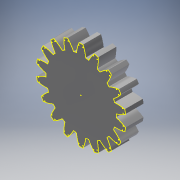
# Autodesk Inventor part: Цилиндрическое зубчатое зацепление1
Saved by Autodesk Inventor 2019 (Build 230136000, 136)
## iProperties
Created: 2020-02-27
Part Number: Цилиндрическое зубчатое зацепление1
Material: Steel
Document SubType Name: Modeling
Designer: Петров Иван
Categories: <?xml version="1.0" encoding="UTF-16"?> <MemberInstance><Categories><FamilyTemplate><FamilyTemplateParameter ValueType="xs:double" Id="1" ObjectReferenceKey="da_z" ObjectType="kUserParameterObject"/><FamilyTemplateParameter ValueType="xs:double" Id="2" ObjectReferenceKey="da_b" ObjectType="kUserParameterObject"/><FamilyTemplateParameter ValueType="xs:double" Id="3" ObjectReferenceKey="da_beta" ObjectType="kUserParameterObject"/><FamilyTemplateParameter ValueType="xs:double" Id="4" ObjectReferenceKey="da_da" ObjectType="kUserParameterObject"/><FamilyTemplateParameter ValueType="xs:double" Id="5" ObjectReferenceKey="da_aw" ObjectType="kUserParameterObject"/><FamilyTemplateParameter ValueType="xs:string" Id="6" ObjectReferenceKey="EAIAABAAAACIAQAAAAAAAIAAAAAAAAAA" ObjectType="83910656" SubObjectId="SurfaceGeometry"/></FamilyTemplate><ParamToTemplateMap><ParamToTemplate CategoryParameter="//CategoryParameter[@InternalName='046C89C9-8512-4d59-83FE-43B91F4F132A']" TemplateParameter="1"/><ParamToTemplate CategoryParameter="//CategoryParameter[@InternalName='2552DF32-E462-4b46-AEBF-C6C7768E72AC']" TemplateParameter="2"/><ParamToTemplate CategoryParameter="//CategoryParameter[@InternalName='C9EE641D-15FC-4fae-A226-E94C4372FDD7']" TemplateParameter="3"/><ParamToTemplate><ParamToTemplate CategoryParameter="//CategoryParameter[@InternalName='00B6519A-459B-49c7-AD84-2E56D39A5744']" ConstantValue="0.000000"/></ParamToTemplate><ParamToTemplate><ParamToTemplate CategoryParameter="//CategoryParameter[@InternalName='04B31F0E-C7A6-4894-AA32-9629BEFACF47']" ConstantValue="1.000000"/></ParamToTemplate><ParamToTemplate><ParamToTemplate CategoryParameter="//CategoryParameter[@InternalName='43CBEC2E-7847-49e7-A936-2F7889FCB2D9']" ConstantValue="0.250000"/></ParamToTemplate><ParamToTemplate><ParamToTemplate CategoryParameter="//CategoryParameter[@InternalName='B1EFC894-105D-4ebd-86BF-FA20ED196853']" ConstantValue="0.350000"/></ParamToTemplate><ParamToTemplate><ParamToTemplate CategoryParameter="//CategoryParameter[@InternalName='51175063-3D10-4879-93E8-6246FE8B403D']" ConstantValue="2060000000.000000"/></ParamToTemplate><ParamToTemplate><ParamToTemplate CategoryParameter="//CategoryParameter[@InternalName='A3A52E27-4454-46a9-B0BD-C932399B70AF']" ConstantValue="0.300000"/></ParamToTemplate><ParamToTemplate><ParamToTemplate CategoryParameter="//CategoryParameter[@InternalName='91B76062-C214-41d9-B1B9-14D2AB99603D']" ConstantValue="0.175000"/></ParamToTemplate><ParamToTemplate><ParamToTemplate CategoryParameter="//CategoryParameter[@InternalName='374E806E-8B8A-4dda-A9AA-1039D6500AD2']" ConstantValue="5.714286"/></ParamToTemplate><ParamToTemplate><ParamToTemplate CategoryParameter="//CategoryParameter[@InternalName='2D373A89-B862-43d6-8D0B-0CBF12AB9F6C']" ConstantValue="0.523599"/></ParamToTemplate><ParamToTemplate CategoryParameter="//CategoryParameter[@InternalName='37777632-D6A2-4fac-9D53-DB8ACD95C989']" TemplateParameter="4"/><ParamToTemplate CategoryParameter="//CategoryParameter[@InternalName='FD1017F1-B727-4f7e-9707-0F86F1FF9423']" TemplateParameter="5"/><ParamToTemplate><ParamToTemplate CategoryParameter="//CategoryParameter[@InternalName='9E1B4470-B2D3-4ff1-B813-535BB4CDF51A']" ConstantValue="3520000.000000"/></ParamToTemplate><ParamToTemplate><ParamToTemplate CategoryParameter="//CategoryParameter[@InternalName='F8452263-BFF6-458c-9FB1-07C4B99E95CD']" ConstantValue="11400000.000000"/></ParamToTemplate><ParamToTemplate><ParamToTemplate CategoryParameter="//CategoryParameter[@InternalName='3E3BB259-FD49-497f-8171-6EBC954A3479']" ConstantValue="2.000000"/></ParamToTemplate><ParamToTemplate CategoryParameter="//CategoryParameter[@InternalName='27C3BAF2-7550-4e4b-AE2C-0DB134B7D9B7']" TemplateParameter="6"/></ParamToTemplateMap><Category DisplayName="Gear" InternalName="DC85795E-93AB-48d5-8EEE-5A27447B64BD" Mnemonic="Gear"><CategoryParameter DisplayName="z" InternalName="046C89C9-8512-4d59-83FE-43B91F4F132A" Mnemonic="z"/><CategoryParameter DisplayName="b" InternalName="2552DF32-E462-4b46-AEBF-C6C7768E72AC" Mnemonic="b"/><CategoryParameter DisplayName="||b|" InternalName="C9EE641D-15FC-4fae-A226-E94C4372FDD7" Mnemonic="beta"/><CategoryParameter DisplayName="x" InternalName="00B6519A-459B-49c7-AD84-2E56D39A5744" Mnemonic="x"/><CategoryParameter DisplayName="a*" InternalName="04B31F0E-C7A6-4894-AA32-9629BEFACF47" Mnemonic="a"/><CategoryParameter DisplayName="c*" InternalName="43CBEC2E-7847-49e7-A936-2F7889FCB2D9" Mnemonic="c"/><CategoryParameter DisplayName="r|.f|*" InternalName="B1EFC894-105D-4ebd-86BF-FA20ED196853" Mnemonic="rf"/><CategoryParameter DisplayName="E" InternalName="51175063-3D10-4879-93E8-6246FE8B403D" Mnemonic="E"/><CategoryParameter DisplayName="||m|" InternalName="A3A52E27-4454-46a9-B0BD-C932399B70AF" Mnemonic="mi"/><Category DisplayName="SpurGear" InternalName="26C5A22E-A91E-4dfd-A3B3-23CCAFAE1764" Mnemonic="SpurGear"><CategoryParameter DisplayName="m" InternalName="91B76062-C214-41d9-B1B9-14D2AB99603D" Mnemonic="m"/><CategoryParameter DisplayName="P" InternalName="374E806E-8B8A-4dda-A9AA-1039D6500AD2" Mnemonic="PP"/><CategoryParameter DisplayName="||a|" InternalName="2D373A89-B862-43d6-8D0B-0CBF12AB9F6C" Mnemonic="alpha"/><CategoryParameter DisplayName="d|.a|" InternalName="37777632-D6A2-4fac-9D53-DB8ACD95C989" Mnemonic="da"/><CategoryParameter DisplayName="a|.w|" InternalName="FD1017F1-B727-4f7e-9707-0F86F1FF9423" Mnemonic="aw"/><CategoryParameter DisplayName="||s||.Flim|" InternalName="9E1B4470-B2D3-4ff1-B813-535BB4CDF51A" Mnemonic="sFlim"/><CategoryParameter DisplayName="||s||.Hlim|" InternalName="F8452263-BFF6-458c-9FB1-07C4B99E95CD" Mnemonic="sHlim"/><CategoryParameter DisplayName="тип" InternalName="3E3BB259-FD49-497f-8171-6EBC954A3479" Mnemonic="type"/><CategoryParameter DisplayName="PitchDiameter" InternalName="27C3BAF2-7550-4e4b-AE2C-0DB134B7D9B7" Mnemonic="IDS_PITCHDIAM"/></Category></Category></Categories></MemberInstance>
Density: 1 g/cm^3
Appearance: Steel
CustomPartVersion: 1
Author: Петров Иван
Autodesk Inventor part; units mm, degrees
ref_plane "YZ Plane" through (0, 0, 0) normal (1, 0, 0) x (0, 1, 0)
ref_plane "XZ Plane" through (0, 0, 0) normal (0, 1, 0) x (-1, 0, 0)
ref_plane "XY Plane" through (0, 0, 0) normal (0, 0, 1) x (1, 0, 0)
sketch "Sketch1" plane through (0, 0, 0) normal (0, 0, 1) x (1, 0, 0)
  circle A0 centre (0, 0) radius 17.3215
  dimension "d0" = 34.6431
  constraints: 1 centre point
  measures "d0" diameter of A0
extrude "Extrusion1" add sketch "Sketch1" along normal blind 7
ref_plane "Work Plane2" through (0, 0, 3.5) normal (0, 0, 1) x (1, 0, 0)
sketch "Sketch2" plane through (0, 0, 0) normal (0, 0, -1) x (-1, 0, 0)
  circle A0 centre (0, 0) radius 17.3215 projected
  circle A1 centre (0, 0) radius 15
  dimension "d3" = 30
  constraints: 1 centre point, 1 coincident
  measures "d3" diameter of A1
surface extrude "Средний диаметр" sketch "Sketch2" against normal through all shown no curves A1
ref_plane "Work Plane8" through (0, 0, 0) normal (0.9848078, 0.1736482, 0) x (0, 0, 1)
ref_plane "Work Plane9" through (0, 0, 0) normal (1, 0, 0) x (0, 1, 0)
spur gear teeth "Цилиндрическое зубчатое зацепление" teeth 18 pitch diameter 31.5 tip diameter 34.6431 root diameter 27.125 face width 7 start plane through (0, 0, 0) normal (0, 0, -1) x (-1, 0, 0)
sketch "Эскиз3" plane through (0, 0, 7) normal (0, 0, 1) x (1, 0, 0)
  arc A0 (-6.6287, 16.003) -> (-6.2625, 12.0301) centre (6.35, 15.196) ccw projected
  arc A1 (-6.2625, 12.0301) -> (-7.2871, 11.4385) centre (0, 0) ccw projected
  arc A2 (-7.2871, 11.4385) -> (-10.5447, 13.7421) centre (-16.3351, 2.0988) ccw projected
  arc A3 (-10.5447, 13.7421) -> (-11.7023, 12.7708) centre (0, 0) ccw projected
  arc A4 (-11.7023, 12.7708) -> (-9.9993, 9.1627) centre (0.7697, 16.4514) ccw projected
  arc A5 (-9.9993, 9.1627) -> (-10.7599, 8.2563) centre (0, 0) ccw projected
  arc A6 (-10.7599, 8.2563) -> (-14.6088, 9.3069) centre (-16.0678, -3.6147) ccw projected
  arc A7 (-14.6088, 9.3069) -> (-15.3644, 7.9982) centre (0, 0) ccw projected
  arc A8 (-15.3644, 7.9982) -> (-12.5301, 5.1901) centre (-4.9034, 15.7225) ccw projected
  arc A9 (-12.5301, 5.1901) -> (-12.9348, 4.0783) centre (0, 0) ccw projected
  arc A10 (-12.9348, 4.0783) -> (-16.911, 3.7491) centre (-13.8625, -8.8922) ccw projected
  arc A11 (-16.911, 3.7491) -> (-17.1734, 2.2609) centre (0, 0) ccw projected
  arc A12 (-17.1734, 2.2609) -> (-13.5496, 0.5916) centre (-9.9851, 13.0972) ccw projected
  arc A13 (-13.5496, 0.5916) -> (-13.5496, -0.5916) centre (0, 0) ccw projected
  arc A14 (-13.5496, -0.5916) -> (-17.1734, -2.2609) centre (-9.9851, -13.0972) ccw projected
  arc A15 (-17.1734, -2.2609) -> (-16.911, -3.7491) centre (0, 0) ccw projected
  arc A16 (-16.911, -3.7491) -> (-12.9348, -4.0783) centre (-13.8625, 8.8922) ccw projected
  arc A17 (-12.9348, -4.0783) -> (-12.5301, -5.1901) centre (0, 0) ccw projected
  arc A18 (-12.5301, -5.1901) -> (-15.3644, -7.9982) centre (-4.9034, -15.7225) ccw projected
  arc A19 (-15.3644, -7.9982) -> (-14.6088, -9.3069) centre (0, 0) ccw projected
  arc A20 (-14.6088, -9.3069) -> (-10.7599, -8.2563) centre (-16.0678, 3.6147) ccw projected
  arc A21 (-10.7599, -8.2563) -> (-9.9993, -9.1627) centre (0, 0) ccw projected
  arc A22 (-9.9993, -9.1627) -> (-11.7023, -12.7708) centre (0.7697, -16.4514) ccw projected
  arc A23 (-11.7023, -12.7708) -> (-10.5447, -13.7421) centre (0, 0) ccw projected
  arc A24 (-10.5447, -13.7421) -> (-7.2871, -11.4385) centre (-16.3351, -2.0988) ccw projected
  arc A25 (-7.2871, -11.4385) -> (-6.2625, -12.0301) centre (0, 0) ccw projected
  arc A26 (-6.2625, -12.0301) -> (-6.6287, -16.003) centre (6.35, -15.196) ccw projected
  arc A27 (-6.6287, -16.003) -> (-5.2087, -16.5199) centre (0, 0) ccw projected
  arc A28 (-5.2087, -16.5199) -> (-2.9355, -13.241) centre (-14.6321, -7.5591) ccw projected
  arc A29 (-2.9355, -13.241) -> (-1.7703, -13.4465) centre (0, 0) ccw projected
  arc A30 (-1.7703, -13.4465) -> (-0.7556, -17.3051) centre (11.1643, -12.1077) ccw projected
  arc A31 (-0.7556, -17.3051) -> (0.7556, -17.3051) centre (0, 0) ccw projected
  arc A32 (0.7556, -17.3051) -> (1.7703, -13.4465) centre (-11.1643, -12.1077) ccw projected
  arc A33 (1.7703, -13.4465) -> (2.9355, -13.241) centre (0, 0) ccw projected
  arc A34 (2.9355, -13.241) -> (5.2087, -16.5199) centre (14.6321, -7.5591) ccw projected
  arc A35 (5.2087, -16.5199) -> (6.6287, -16.003) centre (0, 0) ccw projected
  arc A36 (6.6287, -16.003) -> (6.2625, -12.0301) centre (-6.35, -15.196) ccw projected
  arc A37 (6.2625, -12.0301) -> (7.2871, -11.4385) centre (0, 0) ccw projected
  arc A38 (7.2871, -11.4385) -> (10.5447, -13.7421) centre (16.3351, -2.0988) ccw projected
  arc A39 (10.5447, -13.7421) -> (11.7023, -12.7708) centre (0, 0) ccw projected
  arc A40 (11.7023, -12.7708) -> (9.9993, -9.1627) centre (-0.7697, -16.4514) ccw projected
  arc A41 (9.9993, -9.1627) -> (10.7599, -8.2563) centre (0, 0) ccw projected
  arc A42 (10.7599, -8.2563) -> (14.6088, -9.3069) centre (16.0678, 3.6147) ccw projected
  arc A43 (14.6088, -9.3069) -> (15.3644, -7.9982) centre (0, 0) ccw projected
  arc A44 (15.3644, -7.9982) -> (12.5301, -5.1901) centre (4.9034, -15.7225) ccw projected
  arc A45 (12.5301, -5.1901) -> (12.9348, -4.0783) centre (0, 0) ccw projected
  arc A46 (12.9348, -4.0783) -> (16.911, -3.7491) centre (13.8625, 8.8922) ccw projected
  arc A47 (16.911, -3.7491) -> (17.1734, -2.2609) centre (0, 0) ccw projected
  arc A48 (17.1734, -2.2609) -> (13.5496, -0.5916) centre (9.9851, -13.0972) ccw projected
  arc A49 (13.5496, -0.5916) -> (13.5496, 0.5916) centre (0, 0) ccw projected
  arc A50 (13.5496, 0.5916) -> (17.1734, 2.2609) centre (9.9851, 13.0972) ccw projected
  arc A51 (17.1734, 2.2609) -> (16.911, 3.7491) centre (0, 0) ccw projected
  arc A52 (16.911, 3.7491) -> (12.9348, 4.0783) centre (13.8625, -8.8922) ccw projected
  arc A53 (12.9348, 4.0783) -> (12.5301, 5.1901) centre (0, 0) ccw projected
  arc A54 (12.5301, 5.1901) -> (15.3644, 7.9982) centre (4.9034, 15.7225) ccw projected
  arc A55 (15.3644, 7.9982) -> (14.6088, 9.3069) centre (0, 0) ccw projected
  arc A56 (14.6088, 9.3069) -> (10.7599, 8.2563) centre (16.0678, -3.6147) ccw projected
  arc A57 (10.7599, 8.2563) -> (9.9993, 9.1627) centre (0, 0) ccw projected
  arc A58 (9.9993, 9.1627) -> (11.7023, 12.7708) centre (-0.7697, 16.4514) ccw projected
  arc A59 (11.7023, 12.7708) -> (10.5447, 13.7421) centre (0, 0) ccw projected
  arc A60 (10.5447, 13.7421) -> (7.2871, 11.4385) centre (16.3351, 2.0988) ccw projected
  arc A61 (7.2871, 11.4385) -> (6.2625, 12.0301) centre (0, 0) ccw projected
  arc A62 (6.2625, 12.0301) -> (6.6287, 16.003) centre (-6.35, 15.196) ccw projected
  arc A63 (6.6287, 16.003) -> (5.2087, 16.5199) centre (0, 0) ccw projected
  arc A64 (5.2087, 16.5199) -> (2.9355, 13.241) centre (14.6321, 7.5591) ccw projected
  arc A65 (2.9355, 13.241) -> (1.7703, 13.4465) centre (0, 0) ccw projected
  arc A66 (1.7703, 13.4465) -> (0.7556, 17.3051) centre (-11.1643, 12.1077) ccw projected
  arc A67 (0.7556, 17.3051) -> (-0.7556, 17.3051) centre (0, 0) ccw projected
  arc A68 (-0.7556, 17.3051) -> (-1.7703, 13.4465) centre (11.1643, 12.1077) ccw projected
  arc A69 (-1.7703, 13.4465) -> (-2.9355, 13.241) centre (0, 0) ccw projected
  arc A70 (-2.9355, 13.241) -> (-5.2087, 16.5199) centre (-14.6321, 7.5591) ccw projected
  arc A71 (-5.2087, 16.5199) -> (-6.6287, 16.003) centre (0, 0) ccw projected
equation "\"d0\" = da_da"
equation "\"d1\" = da_b"
equation "\"d3\" = da_dw"
equation "\"d16\" = da_aw"
equation "\"d43\" = da_aw"
equation "\"d46\" = da_aw"
equation "\"da_da\" = 34.643092"
equation "\"da_b\" = 7"
equation "\"da_dw\" = 30"
equation "\"da_aw\" = 45"
body "Solid1"
body "Srf1"
